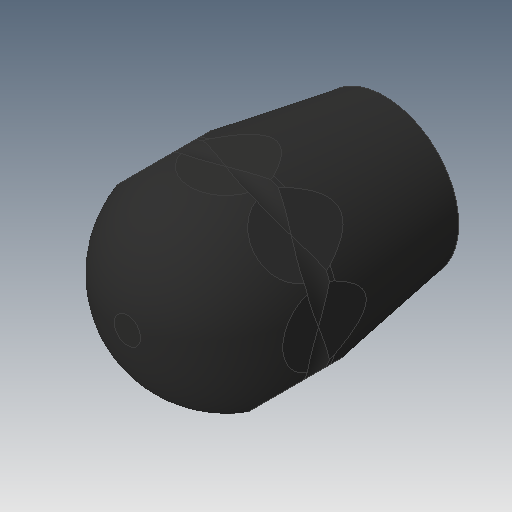
# Autodesk Inventor part: grip_gom
Saved by Autodesk Inventor 2019.4 (Build 234330000, 330)
## iProperties
Created: 2018-02-01
Part Number: grip_gom
Material: ゴム
Document SubType Name: Modeling
Designer: y6tada
Density: 0.93 g/cm^3
Appearance: ゴム - 黒
Mass: 1.34657 g
Surface Area: 13.6732 cm^2
Volume: 1.44792 cm^3
Author: y6tada
Autodesk Inventor part; units mm, degrees
ref_plane "YZ Plane" through (0, 0, 0) normal (1, 0, 0) x (0, 1, 0)
ref_plane "XZ Plane" through (0, 0, 0) normal (0, 1, 0) x (-1, 0, 0)
ref_plane "XY Plane" through (0, 0, 0) normal (0, 0, 1) x (1, 0, 0)
sketch "スケッチ1" plane through (0, 0, 0) normal (1, 0, 0) x (0, 1, 0)
  line L0 (-3.5, 0) -> (-5, 0)
  line L1 (-5, 0) -> (-5, -12)
  line L2 (-5, -12) -> (-5.6, -12)
  line L3 (-5.6, -12) -> (-7.3976, -1.2353)
  arc A0 (0, 7.5) -> (-1, 7.433) centre (0, 0) ccw construction
  line L4 (0, 7.5) -> (0, 7.433) construction
  line L5 (0, 7.433) -> (-1, 7.433)
  arc A1 (-1, 7.433) -> (-7.4531, 0.8372) centre (0, 0) ccw
  line L6 (0, 7.433) -> (0, 3.5)
  arc A2 (-7.4531, -0.8372) -> (-7.4531, 0.8372) centre (-8, 0) ccw
  arc A3 (-7.4531, 0.8372) -> (-7.4531, -0.8372) centre (0, 0) ccw construction
  arc A4 (-7.4531, -0.8372) -> (-7.3976, -1.2353) centre (0, 0) ccw
  arc A5 (0, 3.5) -> (-3.5, 0) centre (0, 0) ccw
  line L7 (0, 0) -> (-3.5, 0) construction
  line L8 (0, 0) -> (0, -5.7661)
  dimension "d2" = 0.6
  dimension "d4" = 7.5
  dimension "d12" = 1
  dimension "d13" = 1
  dimension "d14" = 8
  dimension "d16" = 1.5
  dimension "d17" = 3.5
  dimension "d18" = 12
  constraints: 18 end point, 13 point on circle, 6 centre point, 4 perpendicular, 4 tangent, 3 vertical, 2 coincident, 2 collinear, 1 horizontal, 1 point on line
  measures "d2" distance of L1.end L2.end
  measures "d4" radius of A0
  measures "d12" distance of L4.end L5.end
  measures "d13" radius of A2
  measures "d14" distance of A0.centre A2.centre
  measures "d16" distance of L0.start L0.end
  measures "d17" distance of L0.start L7.start
  measures "d18" distance between parallel lines of L2 L7
revolve "回転1" add sketch "スケッチ1" angle 360 about axis through (0, 0, 0) along (0, 0, -1)
sketch "スケッチ2" plane through (0, 0, 0) normal (0, 0, 1) x (1, 0, 0)
  line L0 (-5.7089, 9.5658) -> (5.7731, 9.5658)
  line L1 (5.7731, 9.5658) -> (5.7731, 7)
  line L2 (5.7731, 7) -> (-5.7089, 7)
  line L3 (-5.7089, 7) -> (-5.7089, 9.5658)
  point P0 (0, 0)
  dimension "d6" = 7
  constraints: 8 end point, 2 parallel, 1 horizontal, 1 perpendicular
  measures "d6" distance from line of point (0, 0) L2
extrude "押し出し1" cut sketch "スケッチ2" along normal mid plane 10
pattern_circular "円形状パターン2" count 8 over 360 about axis through (0, 0, -6) along (0, 0, -1) of "押し出し1"
